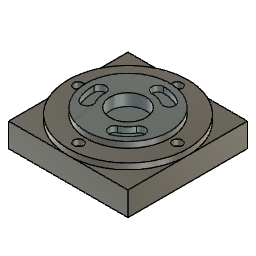
Base Plate 01 (Autodesk Fusion 360 design; units mm, degrees)
Autodesk Fusion 360 part; units mm, degrees
sketch "Sketch1" plane through (0, 0, 0) normal (0, 0, 1) x (1, 0, 0)
  line L0 (50, -50) -> (-50, -50)
  line L1 (-50, -50) -> (-50, 50)
  line L2 (-50, 50) -> (50, 50)
  line L3 (50, 50) -> (50, -50)
  line L4 (50, -50) -> (-50, 50) construction
  line L5 (-50, -50) -> (50, 50) construction
  dimension "d1" = 100
  dimension "d2" = 100
  constraint horizontal L0
  constraint perpendicular L0 L1
  constraint parallel L0 L2
  constraint parallel L1 L3
  constraint coincident L4 origin
  constraint coincident L5 origin
  measures "d1" distance of L0.end L1.end
  measures "d2" distance of L0.start L0.end
extrude "Extrude1" add sketch "Sketch1" along normal blind 20
sketch "Sketch2" plane through (0, 0, 20) normal (0, 0, 1) x (-1, 0, 0)
  line L0 (-50, -50) -> (50, -50)
  line L1 (50, -50) -> (50, 50)
  line L2 (50, 50) -> (-50, 50)
  line L3 (-50, 50) -> (-50, -50)
  circle A0 centre (0, 0) radius 50
  constraint coincident A0.centre origin
  constraint tangent L2 A0
extrude "Extrude2" add sketch "Sketch2" along normal blind 5 contours A0
sketch "Sketch3" plane through (0, 0, 25) normal (0, 0, 1) x (-1, 0, 0)
  circle A0 centre (0, 0) radius 50
  circle A1 centre (0, 0) radius 35
  dimension "d7" = 70
  constraint concentric A0 A1
  measures "d7" diameter of A1
extrude "Extrude3" add sketch "Sketch3" along normal blind 5 contours A1
sketch "Sketch4" plane through (0, 0, 30) normal (0, 0, 1) x (-1, 0, 0)
  circle A0 centre (0, 0) radius 35
  circle A1 centre (0, 0) radius 25 construction
  arc A2 (0, -30) -> (0, -20) centre (0, -25) ccw
  arc A3 (-10.8928, -16.7734) -> (-16.3392, -25.1601) centre (-13.616, -20.9668) ccw
  arc A4 (-10.8928, -16.7734) -> (0, -20) centre (0, 0) ccw
  arc A5 (-16.3392, -25.1601) -> (0, -30) centre (0, 0) ccw
  arc A6 (25.9808, 15) -> (17.3205, 10) centre (21.6506, 12.5) ccw
  arc A7 (19.9726, -1.0467) -> (29.9589, -1.5701) centre (24.9657, -1.3084) ccw
  arc A8 (19.9726, -1.0467) -> (17.3205, 10) centre (0, 0) ccw
  arc A9 (29.9589, -1.5701) -> (25.9808, 15) centre (0, 0) ccw
  arc A10 (-25.9808, 15) -> (-17.3205, 10) centre (-21.6506, 12.5) ccw
  arc A11 (-9.0798, 17.8201) -> (-13.6197, 26.7302) centre (-11.3498, 22.2752) ccw
  arc A12 (-9.0798, 17.8201) -> (-17.3205, 10) centre (0, 0) ccw
  arc A13 (-13.6197, 26.7302) -> (-25.9808, 15) centre (0, 0) ccw
  dimension "d11" = 40
  dimension "d12" = 60
  dimension "d13" = 50
  dimension "d16" = 360
  constraint coincident A0.centre A1.centre
  constraint concentric A1 A5
  constraint coincident A1 A2.centre
  constraint tangent A2 A4
  constraint coincident A1 A3.centre
  constraint tangent A3 A4
  measures "d11" diameter of A4
  measures "d12" diameter of A5
  measures "d13" diameter of A1
extrude "Extrude4" cut sketch "Sketch4" against normal blind 5 contours A2 A3 A4 A5 | A6 A7 A8 A9 | A10 A11 A12 A13
sketch "Sketch5" plane through (0, 0, 30) normal (0, 0, 1) x (-1, 0, 0)
  arc A0 (-13.6197, 26.7302) -> (-25.9808, 15) centre (0, 0) ccw
  arc A1 (-9.0798, 17.8201) -> (-13.6197, 26.7302) centre (-11.3498, 22.2752) ccw
  arc A2 (-9.0798, 17.8201) -> (-17.3205, 10) centre (0, 0) ccw
  arc A3 (-25.9808, 15) -> (-17.3205, 10) centre (-21.6506, 12.5) ccw
  arc A4 (-16.3392, -25.1601) -> (0, -30) centre (0, 0) ccw
  arc A5 (-10.8928, -16.7734) -> (-16.3392, -25.1601) centre (-13.616, -20.9668) ccw
  arc A6 (-10.8928, -16.7734) -> (0, -20) centre (0, 0) ccw
  arc A7 (0, -30) -> (0, -20) centre (0, -25) ccw
  arc A8 (29.9589, -1.5701) -> (25.9808, 15) centre (0, 0) ccw
  arc A9 (19.9726, -1.0467) -> (29.9589, -1.5701) centre (24.9657, -1.3084) ccw
  arc A10 (19.9726, -1.0467) -> (17.3205, 10) centre (0, 0) ccw
  arc A11 (25.9808, 15) -> (17.3205, 10) centre (21.6506, 12.5) ccw
  circle A12 centre (0, 0) radius 35
sketch "Sketch6" plane through (0, 0, 30) normal (0, 0, 1) x (1, 0, 0)
  circle A0 centre (0, 0) radius 15
  dimension "d19" = 30
  constraint coincident A0.centre origin
  measures "d19" diameter of A0
extrude "Extrude5" cut sketch "Sketch6" against normal blind 10
sketch "Sketch7" plane through (0, 0, 25) normal (0, 0, 1) x (-1, 0, 0)
  circle A0 centre (0, 0) radius 35
  circle A1 centre (0, 0) radius 50
  circle A2 centre (0, 0) radius 41.5 construction
  line L0 (0, 0) -> (50, 0) construction
  circle A3 centre (41.5, 0) radius 4
  circle A4 centre (0, 41.5) radius 4
  circle A5 centre (-41.5, 0) radius 4
  circle A6 centre (0, -41.5) radius 4
  dimension "d22" = 83
  dimension "d23" = 8
  dimension "d25" = 360
  constraint concentric A0 A2
  constraint coincident A0.centre A1.centre
  constraint coincident A1 L0.end
  constraint horizontal L0
  constraint coincident A2 A3.centre
  constraint coincident L0 A3.centre
  measures "d22" diameter of A2
  measures "d23" diameter of A3
extrude "Extrude6" cut sketch "Sketch7" against normal blind 5 contours A3 | A4 | A5 | A6
